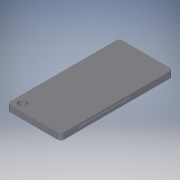
# Autodesk Inventor part: 00_SonyXperiaZ3correct
Saved by Autodesk Inventor 2016 (Build 200138000, 138)
## iProperties
Created: 2016-09-18
Part Number: 00_SonyXperiaZ3correct
Material: Generisch
Document SubType Name: Modeling
Designer: Bene
Density: 1 g/cm^3
Appearance: Vorgabe
Author: Bene
Autodesk Inventor part; units mm, degrees
ref_plane "YZ Plane" through (0, 0, 0) normal (1, 0, 0) x (0, 1, 0)
ref_plane "XZ Plane" through (0, 0, 0) normal (0, 1, 0) x (-1, 0, 0)
ref_plane "XY Plane" through (0, 0, 0) normal (0, 0, 1) x (1, 0, 0)
sketch "Skizze1" plane through (0, 0, 0) normal (0, 0, 1) x (1, 0, 0)
  circle A0 centre (-25, 9.3421) radius 5.1414 projected
  circle A1 centre (-25, 9.3421) radius 4.5
  line L0 (34, -0.6579) -> (-31, -0.6579)
  line L1 (-35, 3.3421) -> (-35, 142.8421)
  line L2 (-31, 146.8421) -> (34, 146.8421)
  line L3 (38, 142.8421) -> (38, 3.3421)
  arc A2 (38, 142.8421) -> (34, 146.8421) centre (34, 142.8421) ccw
  arc A3 (-31, 146.8421) -> (-35, 142.8421) centre (-31, 142.8421) ccw
  arc A4 (-35, 3.3421) -> (-31, -0.6579) centre (-31, 3.3421) ccw
  arc A5 (34, -0.6579) -> (38, 3.3421) centre (34, 3.3421) ccw
  point P0 (0, 0)
  dimension "d0" = 9
  dimension "d1" = 63
  dimension "d2" = 10
  dimension "d3" = 10
  dimension "d4" = 137.5
  dimension "d5" = 4
  constraints: 8 end point, 8 point on circle, 8 tangent, 5 centre point, 3 equal radius, 2 parallel, 1 coincident, 1 horizontal, 1 perpendicular
  measures "d0" diameter of A1
  measures "d1" distance from line of L3 A0.centre
  measures "d2" distance from line of L0 A0.centre
  measures "d3" distance from line of L1 A0.centre
  measures "d4" distance from line of L2 A0.centre
  measures "d5" radius of A2
extrude "Extrusion1" add sketch "Skizze1" along normal blind 8 contours L0 A4 L1 A3 L2 A2 L3 A5
sketch "Skizze2" plane through (38, 3.3421, 0) normal (1, 0, 0) x (0, 0, -1)
  line L0 (0, 0) -> (0, 139.5) projected
  line L1 (0, 139.5) -> (-8, 139.5) projected
  line L2 (-8, 0) -> (-8, 139.5) projected
  line L3 (0, 0) -> (-8, 0) projected
  line L4 (-2.5, 82.5) -> (-5.5, 82.5)
  line L5 (-5.5, 82.5) -> (-5.5, 17.5)
  line L6 (-5.5, 17.5) -> (-2.5, 17.5)
  line L7 (-2.5, 17.5) -> (-2.5, 82.5)
  line L8 (-2.5, 82.5) -> (-5.5, 17.5) construction
  line L9 (-5.5, 82.5) -> (-2.5, 17.5) construction
  point P0 (0, -3.3421)
  point P1 (-4, 50)
  dimension "d8" = 3
  dimension "d9" = 65
  constraints: 12 end point, 2 midpoint, 2 parallel, 1 horizontal, 1 perpendicular
  measures "d8" distance of L6.end L5.end
  measures "d9" distance of L5.end L4.end
extrude "Extrusion2" add sketch "Skizze2" along normal blind 1 contours L7 L6 L5 L4
sketch "Skizze3" plane through (-35, 3.3421, 0) normal (-1, 0, 0) x (0, 0, 1)
  line L0 (0, 139.5) -> (0, 0) projected
  line L1 (0, 0) -> (8, 0) projected
  line L2 (8, 139.5) -> (8, 0) projected
  line L3 (0, 139.5) -> (8, 139.5) projected
  line L4 (2.5, 82.5) -> (2.5, 17.5) projected
  line L5 (5.5, 92.5) -> (2.5, 92.5)
  line L6 (2.5, 92.5) -> (2.5, 42.5)
  line L7 (2.5, 42.5) -> (5.5, 42.5)
  line L8 (5.5, 42.5) -> (5.5, 92.5)
  line L9 (5.5, 92.5) -> (2.5, 42.5) construction
  line L10 (2.5, 92.5) -> (5.5, 42.5) construction
  line L11 (5.5, 135.0516) -> (2.5, 135.0516)
  line L12 (2.5, 135.0516) -> (2.5, 116.0593)
  line L13 (2.5, 116.0593) -> (5.5, 116.0593)
  line L14 (5.5, 116.0593) -> (5.5, 135.0516)
  line L15 (5.5, 135.0516) -> (2.5, 116.0593) construction
  line L16 (2.5, 135.0516) -> (5.5, 116.0593) construction
  point P0 (0, -3.3421)
  point P1 (4, 67.5)
  point P2 (4, 125.5555)
  dimension "d12" = 50
  constraints: 24 end point, 4 midpoint, 4 parallel, 2 horizontal, 2 perpendicular, 1 point on line
  measures "d12" distance of L6.end L5.end
extrude "Extrusion3" add sketch "Skizze3" along normal blind 1 contours L6 L5 L8 L7 L4 | L14 L13 L12 L11
